# Autodesk Inventor part: ATMEGA328P_TQFP
Saved by Autodesk Inventor 2016 (Build 200138000, 138)
## iProperties
Created: 2016-04-08
Part Number: ATMEGA328P_TQFP
Material: Generic
Document SubType Name: Modeling
Designer: Paschalis
Density: 1 g/cm^3
Appearance: TQFP32-08, ATMEGA328P_TQFP
Author: Paschalis
Autodesk Inventor part; units mm, degrees
ref_plane "YZ Plane" through (0, 0, 0) normal (1, 0, 0) x (0, 1, 0)
ref_plane "XZ Plane" through (0, 0, 0) normal (0, 1, 0) x (-1, 0, 0)
ref_plane "XY Plane" through (0, 0, 0) normal (0, 0, 1) x (1, 0, 0)
sketch "TQFP32-08, ATMEGA328P_TQFP_11" plane through (0, 0, 0) normal (0, 0, 1) x (1, 0, 0)
  line L0 (-4.5466, 4.5466) -> (4.5466, 4.5466)
  line L1 (4.5466, 4.5466) -> (4.5466, -4.5466)
  line L2 (4.5466, -4.5466) -> (-4.5466, -4.5466)
  line L3 (-4.5466, -4.5466) -> (-4.5466, 4.5466)
  constraints: 8 end point
extrude "Extrusion1" add sketch "TQFP32-08, ATMEGA328P_TQFP_11" along normal blind 1
body "Solid1"
